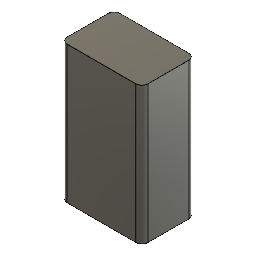
battery_export_fusion (Autodesk Fusion 360 archive; units mm, degrees)
design "02_battery_base"
Autodesk Fusion 360 part; units mm, degrees
sketch "Sketch2" plane through (0, 0, 0) normal (0, 1, 0) x (1, 0, 0)
  line L0 (0, 11) -> (26.3, 11)
  line L1 (26.3, 11) -> (26.3, -6.28)
  line L2 (26.3, -6.28) -> (0, -6.28)
  line L3 (0, -6.28) -> (0, 11)
  line L4 (0, 2.36) -> (3.77, 2.36) construction
  line L5 (3.77, 2.36) -> (9.35, 2.36) construction
  line L6 (9.35, 2.36) -> (16.56, 2.36) construction
  line L7 (16.56, 2.36) -> (23.33, 2.36) construction
  line L8 (23.33, 2.36) -> (26.3, 2.36) construction
  dimension "d8" = 26.3
  dimension "d9" = 17.28
  dimension "d10" = 3.77
  dimension "d11" = 5.58
  dimension "d12" = 7.21
  dimension "d13" = 6.77
  dimension "d14" = 2.97
  constraint horizontal L0
  constraint vertical L1
  constraint horizontal L2
  constraint vertical L3
  constraint midpoint L3 L4.start
  constraint perpendicular L3 L4
  constraint parallel L4 L5
  constraint parallel L5 L6
  constraint parallel L6 L7
  constraint perpendicular L1 L8
  measures "d8" distance of L0.start L0.end
  measures "d9" distance of L0.start L2.end
  measures "d10" distance of L4.start L4.end
  measures "d11" distance of L4.end L5.end
  measures "d12" distance of L5.end L6.end
  measures "d13" distance of L6.end L7.end
  measures "d14" distance of L7.end L8.end
extrude "Extrude1" add sketch "Sketch2" along normal blind 44.67
fillet "Fillet1" radius 2 4 edges at (26.3, 22.335, 6.28) (26.3, 22.335, -11) (0, 22.335, -11) (0, 22.335, 6.28)

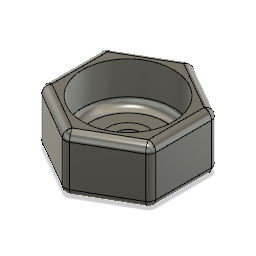
design "02_battery_terminal_negative"
Autodesk Fusion 360 part; units mm, degrees
sketch "Sketch4" plane through (0, 0, 0) normal (0, 1, 0) x (1, 0, 0)
  line L0 (0, 0) -> (6.77, 0) construction
  line L1 (3.385, 1.9543) -> (0, 3.9087)
  line L2 (0, 3.9087) -> (-3.385, 1.9543)
  line L3 (-3.385, 1.9543) -> (-3.385, -1.9543)
  line L4 (-3.385, -1.9543) -> (0, -3.9087)
  line L5 (0, -3.9087) -> (3.385, -1.9543)
  line L6 (3.385, -1.9543) -> (3.385, 1.9543)
  dimension "d28" = 6.77
  constraint coincident L0.start origin
  constraint horizontal L0
  measures "d28" distance of L0.start L0.end
extrude "Extrude3" add sketch "Sketch4" along normal blind 3.4
fillet "Fillet6" radius 0.45 18 edges at (3.385, 3.4, 0) (3.385, 1.7, 1.9543) (1.6925, 3.4, 2.9315) (3.385, 1.7, -1.9543) (1.6925, 3.4, -2.9315) (0, 1.7, -3.9087) (-1.6925, 3.4, -2.9315) (-3.385, 1.7, -1.9543) (-3.385, 3.4, 0) (-3.385, 1.7, 1.9543) (-1.6925, 3.4, 2.9315) (0, 1.7, 3.9087) (1.6925, 0, 2.9315) (-1.6925, 0, 2.9315) (3.385, 0, 0) (1.6925, 0, -2.9315) (-1.6925, 0, -2.9315) (-3.385, 0, 0)
hole "Hole4" at (0, 3.4, 0) direction (0, -1, 0) diameter 5.5 depth 2.5 tip angle 180
fillet "Fillet7" radius 0.5 1 edges at (0.9944, 0.9, -2.5639)
hole "Hole5" at (0, 0.9, 0) direction (0, -1, 0) diameter 2.5 depth 0.1 tip angle 180
extrude "Extrude4" add 1 faces at (-0.4642, 0.8, -0.4866) along direction (0, 1, 0) blind 0.3
hole "Hole6" at (0, 1.1, 0) direction (0, -1, 0) diameter 1.5 depth 0.5 tip angle 180
fillet "Fillet8" radius 0.5 1 edges at (0.2712, 0.6, -0.6992)
